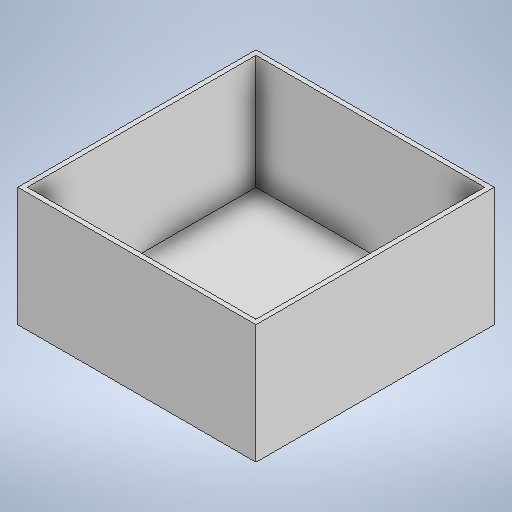
# Autodesk Inventor part: Box
Saved by Autodesk Inventor 2025.2 (Build 292293000, 293)
## iProperties
Created: 2026-07-08
Part Number: Box
Material: Generic
Document SubType Name: Modeling
Designer: Simon
Density: 1 g/cm^3
Appearance: Default
Author: Simon
Autodesk Inventor part; units mm, degrees
ref_plane "YZ Plane" through (0, 0, 0) normal (1, 0, 0) x (0, 1, 0)
ref_plane "XZ Plane" through (0, 0, 0) normal (0, 1, 0) x (-1, 0, 0)
ref_plane "XY Plane" through (0, 0, 0) normal (0, 0, 1) x (1, 0, 0)
sketch "Sketch1" plane through (0, 0, 0) normal (0, 1, 0) x (-1, 0, 0)
  line L0 (0, 0) -> (100, 0)
  line L1 (100, 0) -> (100, -100)
  line L2 (100, -100) -> (0, -100)
  line L3 (0, -100) -> (0, 0)
  line L4 (100, 0) -> (98, 0)
  line L5 (98, 0) -> (98, -2)
  line L6 (98, -2) -> (100, -2)
  line L7 (100, -2) -> (100, 0)
  line L8 (100, -100) -> (98, -100)
  line L9 (98, -100) -> (98, -98)
  line L10 (98, -98) -> (100, -98)
  line L11 (100, -98) -> (100, -100)
  line L12 (0, -100) -> (2, -100)
  line L13 (2, -100) -> (2, -98)
  line L14 (2, -98) -> (0, -98)
  line L15 (0, -98) -> (0, -100)
  line L16 (0, 0) -> (2, 0)
  line L17 (2, 0) -> (2, -2)
  line L18 (2, -2) -> (0, -2)
  line L19 (0, -2) -> (0, 0)
  line L20 (98, -2) -> (2, -2)
  line L21 (2, -2) -> (2, -98)
  line L22 (2, -98) -> (98, -98)
  line L23 (98, -98) -> (98, -2)
  dimension "d0" = 100
  dimension "d1" = 100
  dimension "d2" = 2
  dimension "d3" = 2
  dimension "d4" = 2
  dimension "d5" = 2
  dimension "d6" = 2
  dimension "d7" = 2
  dimension "d8" = 2
  dimension "d9" = 2
  constraints: 48 end point, 12 parallel, 6 horizontal, 6 perpendicular
  measures "d0" distance of L1.end L2.end
  measures "d1" distance of L0.end L1.end
  measures "d2" distance of L6.end L5.end
  measures "d3" distance of L5.end L4.end
  measures "d4" distance of L9.end L10.end
  measures "d5" distance of L8.end L9.end
  measures "d6" distance of L14.end L13.end
  measures "d7" distance of L13.end L12.end
  measures "d8" distance of L17.end L18.end
  measures "d9" distance of L16.end L17.end
extrude "Extrusion1" add sketch "Sketch1" against normal blind 48 contours L0 L17 L18 L3 | L0 L5 L20 L17 | L18 L21 L14 L3 | L0 L1 L6 L5 | L14 L13 L2 L3 | L6 L1 L10 L23 | L22 L9 L2 L13 | L10 L1 L2 L9
sketch "Sketch2" plane through (0, -48, 0) normal (0, -1, 0) x (1, 0, 0)
  line L0 (0, 0) -> (-100, 0)
  line L1 (-100, 0) -> (-100, -100)
  line L2 (-100, -100) -> (0, -100)
  line L3 (0, -100) -> (0, 0)
  constraints: 8 end point, 2 parallel, 1 horizontal, 1 perpendicular
extrude "Extrusion2" add sketch "Sketch2" along normal blind 2
extrude "Extrusion3" [suppressed]
sketch "Sketch4" plane through (0, 48, 0) normal (0, 1, 0) x (1, 0, 0)
  line L0 (-100, 100) -> (0, 100)
  line L1 (0, 100) -> (0, 0)
  line L2 (0, 0) -> (-100, 0)
  line L3 (-100, 0) -> (-100, 100)
  constraints: 8 end point, 2 parallel, 1 horizontal, 1 perpendicular
extrude "Extrusion4" [suppressed]
body "Solid1"
